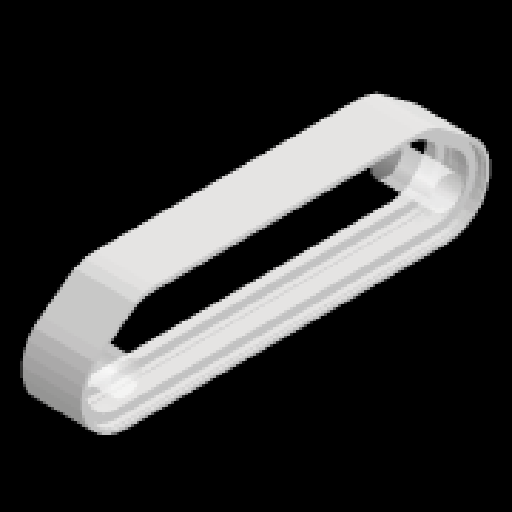
# Autodesk Inventor part: trackplaceholder
Saved by Autodesk Inventor 2023 (Build 270158030, 158C)
## iProperties
Created: 2022-11-20
Part Number: trackplaceholder
Material: Generic
Document SubType Name: Modeling
Designer: kumpu
Density: 1 g/cm^3
Appearance: Default
Author: kumpu
Autodesk Inventor part; units mm, degrees
ref_plane "YZ Plane" through (0, 0, 0) normal (1, 0, 0) x (0, 1, 0)
ref_plane "XZ Plane" through (0, 0, 0) normal (0, 1, 0) x (-1, 0, 0)
ref_plane "XY Plane" through (0, 0, 0) normal (0, 0, 1) x (1, 0, 0)
sketch "Sketch1" plane through (0, 0, 0) normal (0, 0, 1) x (1, 0, 0)
  line L0 (-33.75, -7.3) -> (-33.75, 5.9)
  line L1 (-33.75, 5.9) -> (-17.05, 5.9)
  line L2 (-17.05, 5.9) -> (-17.05, -7.3)
  line L3 (-17.05, -7.3) -> (-7.2, -7.3)
  line L4 (-7.2, -7.3) -> (-7.2, -8.9)
  line L5 (-7.2, -8.9) -> (0, -8.9)
  line L6 (0, -8.9) -> (0, -15.25)
  line L7 (0, -15.25) -> (-47.625, -15.25)
  line L8 (-47.625, -15.25) -> (-47.625, -8.9)
  line L9 (-47.625, -8.9) -> (-43.6, -8.9)
  line L10 (-43.6, -8.9) -> (-43.6, -7.3)
  line L11 (-43.6, -7.3) -> (-33.75, -7.3)
  line L12 (-33.75, 0) -> (-17.05, 0) construction
  line L13 (33.75, -7.3) -> (33.75, 5.9)
  line L14 (33.75, 5.9) -> (17.05, 5.9)
  line L15 (17.05, 5.9) -> (17.05, -7.3)
  line L16 (17.05, -7.3) -> (7.2, -7.3)
  line L17 (7.2, -7.3) -> (7.2, -8.9)
  line L18 (7.2, -8.9) -> (0, -8.9)
  line L19 (0, -15.25) -> (47.625, -15.25)
  line L20 (47.625, -15.25) -> (47.625, -8.9)
  line L21 (47.625, -8.9) -> (43.6, -8.9)
  line L22 (43.6, -8.9) -> (43.6, -7.3)
  line L23 (43.6, -7.3) -> (33.75, -7.3)
  line L24 (33.75, 0) -> (17.05, 0) construction
  point P0 (0, 0)
  point P1 (-25.4, 5.9)
  point P2 (25.4, 5.9)
  dimension "d0" = 6.35
  dimension "d1" = 8.9
  dimension "d2" = 5.9
  dimension "d3" = 1.6
  dimension "d4" = 36.4
  dimension "d5" = 25.4
  dimension "d6" = 16.7
  dimension "d7" = 47.625
  constraints: 50 end point, 13 symmetric about line, 12 point on line, 11 perpendicular, 1 collinear, 1 midpoint, 1 vertical
  measures "d0" distance of L5.end L6.end
  measures "d1" distance between parallel lines of L5 L12
  measures "d2" distance between parallel lines of L12 L1
  measures "d3" distance of L3.end L4.end
  measures "d4" distance between parallel lines of L10 L4
  measures "d5" horizontal distance of point (0, 0) point (-25.4, 5.9)
  measures "d6" distance of L0.end L1.end
  measures "d7" distance between parallel lines of L6 L8
sketch "Sketch2" plane through (0, 0, 0) normal (1, 0, 0) x (0, 1, 0)
  line L0 (0, 254) -> (0, -254) construction
  arc A0 (0, -254) -> (101.8382, -281.7414) centre (54.6976, -254) ccw construction
  line L1 (101.8382, -281.7414) -> (139.1861, -218.2765) construction
  arc A1 (139.1861, -218.2765) -> (143.9286, -200.867) centre (109.6025, -200.867) ccw construction
  line L2 (143.9286, -200.867) -> (143.9286, 218.0085) construction
  arc A2 (143.9286, 218.0085) -> (139.8261, 234.2816) centre (109.6025, 218.0085) ccw construction
  line L3 (12.7968, 218.8411) -> (5.818, 229.4518) construction
  line L4 (5.818, 229.4518) -> (1.4744, 241.3859) construction
  line L5 (1.4744, 241.3859) -> (0, 254) construction
  line L6 (0, 254) -> (1.4744, 266.6141)
  line L7 (1.4744, 266.6141) -> (5.818, 278.5482)
  line L8 (5.818, 278.5482) -> (12.7968, 289.1589)
  line L9 (12.7968, 289.1589) -> (22.0344, 297.8742)
  line L10 (22.0344, 297.8742) -> (33.033, 304.2242)
  line L11 (33.033, 304.2242) -> (45.1994, 307.8666)
  line L12 (45.1994, 307.8666) -> (57.8779, 308.605)
  line L13 (57.8779, 308.605) -> (70.385, 306.3997)
  line L14 (70.385, 306.3997) -> (82.0464, 301.3695)
  line L15 (82.0464, 301.3695) -> (92.2333, 293.7856)
  line L16 (92.2333, 293.7856) -> (100.3967, 284.0568)
  line L17 (100.3967, 284.0568) -> (106.0965, 272.7077) construction
  line L18 (106.0965, 272.7077) -> (109.0253, 260.35) construction
  line L19 (109.0253, 260.35) -> (109.0253, 247.65) construction
  line L20 (109.0253, 247.65) -> (106.0965, 235.2923) construction
  line L21 (106.0965, 235.2923) -> (100.3967, 223.9432) construction
  line L22 (100.3967, 223.9432) -> (92.2333, 214.2144) construction
  line L23 (92.2333, 214.2144) -> (82.0464, 206.6305) construction
  line L24 (82.0464, 206.6305) -> (70.385, 201.6003) construction
  line L25 (70.385, 201.6003) -> (57.8779, 199.395) construction
  line L26 (57.8779, 199.395) -> (45.1994, 200.1334) construction
  line L27 (45.1994, 200.1334) -> (33.033, 203.7758) construction
  line L28 (33.033, 203.7758) -> (22.0344, 210.1258) construction
  line L29 (22.0344, 210.1258) -> (12.7968, 218.8411) construction
  line L30 (54.6976, 254) -> (0, 254) construction
  arc A3 (100.3967, 284.0568) -> (0, 254) centre (54.6976, 254) ccw construction
  line L31 (139.8261, 234.2816) -> (100.3967, 284.0568)
  line L32 (143.6743, 222.1786) -> (139.8261, 234.2816)
  line L33 (0, 0) -> (173.098, 0) construction
  line L34 (143.9286, 196.85) -> (143.9286, 0)
  line L35 (0, 254) -> (0, 0)
  line L36 (0, 0) -> (143.9286, 0) construction
  arc A4 (139.8261, -234.2816) -> (143.9286, -218.0085) centre (109.6025, -218.0085) ccw construction
  line L37 (12.7968, -218.8411) -> (5.818, -229.4518) construction
  line L38 (5.818, -229.4518) -> (1.4744, -241.3859) construction
  line L39 (1.4744, -241.3859) -> (0, -254) construction
  line L40 (0, -254) -> (1.4744, -266.6141)
  line L41 (1.4744, -266.6141) -> (5.818, -278.5482)
  line L42 (5.818, -278.5482) -> (12.7968, -289.1589)
  line L43 (12.7968, -289.1589) -> (22.0344, -297.8742)
  line L44 (22.0344, -297.8742) -> (33.033, -304.2242)
  line L45 (33.033, -304.2242) -> (45.1994, -307.8666)
  line L46 (45.1994, -307.8666) -> (57.8779, -308.605)
  line L47 (57.8779, -308.605) -> (70.385, -306.3997)
  line L48 (70.385, -306.3997) -> (82.0464, -301.3695)
  line L49 (82.0464, -301.3695) -> (92.2333, -293.7856)
  line L50 (92.2333, -293.7856) -> (100.3967, -284.0568)
  line L51 (100.3967, -284.0568) -> (106.0965, -272.7077) construction
  line L52 (106.0965, -272.7077) -> (109.0253, -260.35) construction
  line L53 (109.0253, -260.35) -> (109.0253, -247.65) construction
  line L54 (109.0253, -247.65) -> (106.0965, -235.2923) construction
  line L55 (106.0965, -235.2923) -> (100.3967, -223.9432) construction
  line L56 (100.3967, -223.9432) -> (92.2333, -214.2144) construction
  line L57 (92.2333, -214.2144) -> (82.0464, -206.6305) construction
  line L58 (82.0464, -206.6305) -> (70.385, -201.6003) construction
  line L59 (70.385, -201.6003) -> (57.8779, -199.395) construction
  line L60 (57.8779, -199.395) -> (45.1994, -200.1334) construction
  line L61 (45.1994, -200.1334) -> (33.033, -203.7758) construction
  line L62 (33.033, -203.7758) -> (22.0344, -210.1258) construction
  line L63 (22.0344, -210.1258) -> (12.7968, -218.8411) construction
  line L64 (54.6976, -254) -> (0, -254) construction
  line L65 (142.8586, -209.5048) -> (143.6743, -222.1786)
  arc A5 (0, -254) -> (100.3967, -284.0568) centre (54.6976, -254) ccw construction
  line L66 (139.8261, -234.2816) -> (100.3967, -284.0568)
  line L67 (143.6743, -222.1786) -> (139.8261, -234.2816)
  line L68 (142.8586, -209.5048) -> (143.9286, -196.85)
  line L69 (143.9286, -196.85) -> (143.9286, 0)
  line L70 (0, -254) -> (0, 0)
  line L71 (143.6743, 222.1786) -> (144.7443, 209.5238)
  line L72 (144.7443, 209.5238) -> (143.9286, 196.85)
  dimension "d9" = 12.7
  dimension "d12" = 508
  dimension "d19" = 63.5
  dimension "d20" = 89.231
  dimension "d22" = 196.85
  constraints: 146 end point, 35 symmetric about line, 15 point on circle, 6 centre point, 6 coincident, 5 equal length, 5 tangent, 3 horizontal, 3 point on line, 3 vertical, 2 equal radius, 1 midpoint, 1 parallel, 57 other
  measures "d9" distance of L19.end L20.end
  measures "d12" distance of L0.start L0.end
  measures "d19" distance of L31.start L31.end
  measures "d20" distance from line of L30.start L2
  measures "d22" distance from line of L33 L34.start
sweep "Sweep1" add profiles "Sketch1" path "Sketch2" path curves L70 L40 L41 L42 L43 L44 L45 L46 L47 L48 L49 L50 L66 L67 L65 L68 L69 L34 L72 L71 L32 L31 L16 L15 L14 L13 L12 L11 L10 L9 L8 L7 L6 L35
sketch "Sketch3" plane through (47.625, -15.25, -254.8882) normal (-1, 0, 0) x (0, 0, 1)
  circle A0 centre (0.8882, 69.9476) radius 70.0514 construction
  circle A1 centre (508.9687, 69.9717) radius 69.9763 construction
  circle A2 centre (0.8882, 69.9476) radius 25.4
  circle A3 centre (508.9687, 69.9717) radius 25.4
  point P0 (254.8882, 15.25)
  point P1 (-59.7781, 104.9733)
  point P2 (-63.4341, 42.2016)
  point P3 (-30.5508, 7.3474)
  point P4 (559.8417, 118.0197)
  point P5 (577.8754, 57.7833)
  point P6 (509.7764, 0)
  dimension "d14" = 50.8
  dimension "d15" = 50.8
  constraints: 6 point on circle, 4 centre point, 2 coincident
  measures "d14" diameter of A2
  measures "d15" diameter of A3
surface extrude "ExtrusionSrf1" sketch "Sketch3" along normal blind 95.25 shown yes curves A2
mirror "Mirror1" about plane through (0, 0, 0) normal (0, 0, 1) of "ExtrusionSrf1"
body "Solid1"
body "Srf1"
body "Srf2"
